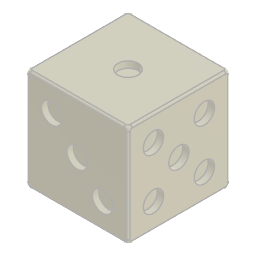
DICE (Autodesk Fusion 360 design; units mm, degrees)
part number: 2026-03-10-20-25-13-652
Autodesk Fusion 360 part; units mm, degrees
sketch "Sketch1" plane through (0, 0, 0) normal (0, 0, 1) x (1, 0, 0)
  line L0 (50.8, -50.8) -> (-50.8, -50.8)
  line L1 (-50.8, -50.8) -> (-50.8, 50.8)
  line L2 (-50.8, 50.8) -> (50.8, 50.8)
  line L3 (50.8, 50.8) -> (50.8, -50.8)
  line L4 (50.8, -50.8) -> (-50.8, 50.8) construction
  line L5 (-50.8, -50.8) -> (50.8, 50.8) construction
  dimension "d1" = 101.6
  dimension "d2" = 101.6
  constraint horizontal L0
  constraint perpendicular L0 L1
  constraint parallel L0 L2
  constraint parallel L1 L3
  constraint coincident L4 origin
  constraint coincident L5 origin
  measures "d1" distance of L1.end L2.end
  measures "d2" distance of L0.end L1.end
extrude "Extrude1" add sketch "Sketch1" along normal mid plane 101.6
sketch "Sketch2" plane through (0, 0, 50.8) normal (0, 0, 1) x (-1, 0, 0)
  line L0 (-50.8, -50.8) -> (50.8, -50.8)
  line L1 (50.8, -50.8) -> (50.8, 50.8)
  line L2 (50.8, 50.8) -> (-50.8, 50.8)
  line L3 (-50.8, 50.8) -> (-50.8, -50.8)
  circle A0 centre (0, 0) radius 10.16
  dimension "d5" = 20.32
  constraint coincident A0.centre origin
  measures "d5" diameter of A0
extrude "Extrude2" cut sketch "Sketch2" against normal blind 6.35 contours A0
sketch "Sketch3" plane through (0, -50.8, 0) normal (0, -1, 0) x (1, 0, 0)
  line L0 (50.8, -50.8) -> (50.8, 50.8)
  line L1 (50.8, 50.8) -> (-50.8, 50.8)
  line L2 (-50.8, 50.8) -> (-50.8, -50.8)
  line L3 (-50.8, -50.8) -> (50.8, -50.8)
  line L4 (-50.8, 50.8) -> (50.8, -50.8) construction
  line L5 (50.8, 50.8) -> (-50.8, -50.8) construction
  circle A0 centre (0, 0) radius 10.16
  circle A1 centre (-25.4, 25.4) radius 10.16
  circle A2 centre (25.4, -25.4) radius 10.16
  dimension "d9" = 20.32
  dimension "d12" = 20.32
  dimension "d13" = 20.32
  constraint coincident L1.end L2.start
  constraint coincident L0.start L3.end
  constraint coincident L0.end L1.start
  constraint coincident L2.end L3.start
  constraint coincident A0.centre origin
  constraint coincident L4 A1.centre
  constraint coincident L4 A2.centre
  measures "d9" diameter of A0
  measures "d12" diameter of A1
  measures "d13" diameter of A2
extrude "Extrude3" cut sketch "Sketch3" against normal blind 6.35 contours A0 | A1 | A2
sketch "Sketch4" plane through (50.8, 0, 0) normal (1, 0, 0) x (0, 1, 0)
  line L0 (50.8, -50.8) -> (50.8, 50.8)
  line L1 (50.8, 50.8) -> (-50.8, 50.8)
  line L2 (-50.8, 50.8) -> (-50.8, -50.8)
  line L3 (-50.8, -50.8) -> (50.8, -50.8)
  line L4 (-50.8, 50.8) -> (50.8, -50.8) construction
  line L5 (50.8, 50.8) -> (-50.8, -50.8) construction
  circle A0 centre (0, 0) radius 10.16
  circle A1 centre (25.4, 25.4) radius 10.16
  circle A2 centre (25.4, -25.4) radius 10.16
  circle A3 centre (-25.4, -25.4) radius 10.16
  circle A4 centre (-25.4, 25.4) radius 10.16
  dimension "d16" = 20.32
  dimension "d17" = 20.32
  dimension "d18" = 20.32
  dimension "d19" = 20.32
  dimension "d20" = 20.32
  constraint coincident L1.end L2.start
  constraint coincident L0.start L3.end
  constraint coincident L0.end L1.start
  constraint coincident L2.end L3.start
  constraint coincident A0.centre origin
  constraint coincident L5 A1.centre
  constraint coincident L4 A2.centre
  constraint coincident L5 A3.centre
  constraint coincident L4 A4.centre
  measures "d16" diameter of A0
  measures "d17" diameter of A1
  measures "d18" diameter of A2
  measures "d19" diameter of A3
  measures "d20" diameter of A4
extrude "Extrude4" cut sketch "Sketch4" against normal blind 6.35 contours A0 | A1 | A2 | A3 | A4
sketch "Sketch5" plane through (0, 50.8, 0) normal (0, 1, 0) x (-1, 0, 0)
  line L0 (50.8, -50.8) -> (50.8, 50.8)
  line L1 (50.8, 50.8) -> (-50.8, 50.8)
  line L2 (-50.8, 50.8) -> (-50.8, -50.8)
  line L3 (-50.8, -50.8) -> (50.8, -50.8)
  circle A0 centre (-25.4, 25.4) radius 10.16
  circle A1 centre (25.4, 25.4) radius 10.16
  circle A2 centre (25.4, -25.4) radius 10.16
  circle A3 centre (-25.4, -25.4) radius 10.16
  dimension "d26" = 20.32
  constraint equal A0 A1
  constraint equal A0 A2
  constraint equal A0 A3
  measures "d26" diameter of A0
extrude "Extrude5" cut sketch "Sketch5" against normal blind 6.35 contours A0 | A1 | A2 | A3
sketch "Sketch6" plane through (-50.8, 0, 0) normal (-1, 0, 0) x (0, -1, 0)
  line L0 (50.8, -50.8) -> (50.8, 50.8)
  line L1 (50.8, 50.8) -> (-50.8, 50.8)
  line L2 (-50.8, 50.8) -> (-50.8, -50.8)
  line L3 (-50.8, -50.8) -> (50.8, -50.8)
  circle A0 centre (-25.4, 25.4) radius 10.16
  circle A1 centre (25.4, -25.4) radius 10.16
  dimension "d29" = 20.32
  dimension "d30" = 20.32
  measures "d29" diameter of A0
  measures "d30" diameter of A1
extrude "Extrude6" cut sketch "Sketch6" against normal blind 6.35 contours A0 | A1
sketch "Sketch7" plane through (0, 0, -50.8) normal (0, 0, -1) x (1, 0, 0)
  line L0 (-50.8, -50.8) -> (50.8, -50.8)
  line L1 (50.8, -50.8) -> (50.8, 50.8)
  line L2 (50.8, 50.8) -> (-50.8, 50.8)
  line L3 (-50.8, 50.8) -> (-50.8, -50.8)
  circle A0 centre (-25.4, 0) radius 10.16
  circle A1 centre (-25.4, -25.4) radius 10.16
  circle A2 centre (-25.4, 25.4) radius 10.16
  circle A3 centre (25.4, 25.4) radius 10.16
  circle A4 centre (25.4, 0) radius 10.16
  circle A5 centre (25.4, -25.4) radius 10.16
  dimension "d33" = 20.32
  constraint equal A0 A2
  constraint equal A0 A3
  constraint equal A0 A4
  constraint equal A1 A5
  constraint equal A4 A5
  measures "d33" diameter of A0
extrude "Extrude7" cut sketch "Sketch7" against normal blind 6.35 contours A0 | A1 | A2 | A3 | A4 | A5
fillet "Fillet1" radius 2.032 12 edges at (50.8, 0, 50.8) (0, 50.8, 50.8) (-50.8, 0, 50.8) (0, -50.8, 50.8) (-50.8, -50.8, 0) (50.8, -50.8, 0) (50.8, 50.8, 0) (-50.8, 50.8, 0) (0, 50.8, -50.8) (50.8, 0, -50.8) (0, -50.8, -50.8) (-50.8, 0, -50.8)
equation "d1 = dicesize"
equation "d2 = dicesize"
equation "d3 = dicesize / 2"
equation "d5 = DivotDia"
equation "d6 = ( -1 / 4 ) * 1 in"
equation "d9 = DivotDia"
equation "d12 = DivotDia"
equation "d13 = DivotDia"
equation "d14 = ( -1 / 4 ) * 1 in"
equation "d16 = DivotDia"
equation "d17 = DivotDia"
equation "d18 = DivotDia"
equation "d19 = DivotDia"
equation "d20 = DivotDia"
equation "d21 = ( -1 / 4 ) * 1 in"
equation "dicesize = 4 in"
equation "DivotDia = 0.8 in"
equation "DivotDepth = 0.25 in"
equation "d26 = DivotDia"
equation "d27 = -DivotDepth"
equation "d29 = DivotDia"
equation "d30 = DivotDia"
equation "d31 = -DivotDepth"
equation "d33 = DivotDia"
equation "d34 = -DivotDepth"
